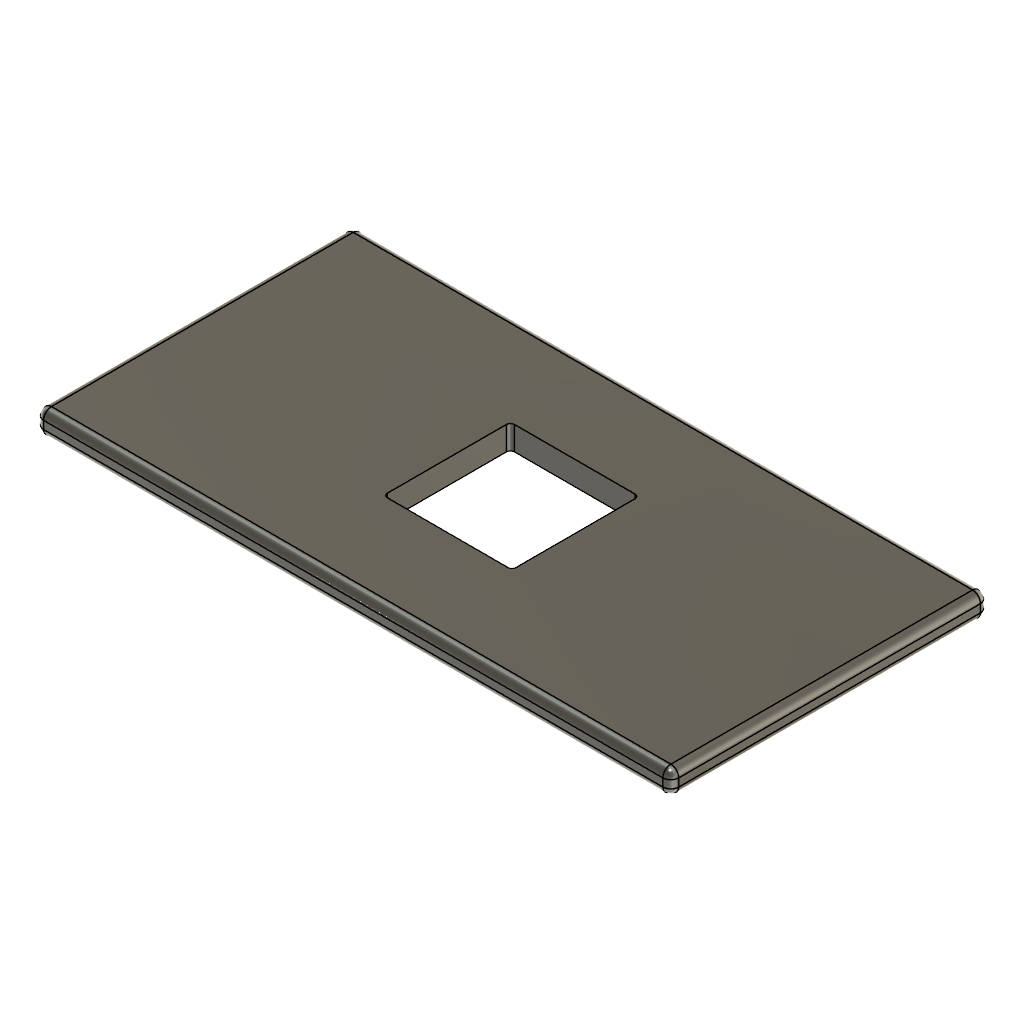
Fan_Holder (Autodesk Fusion 360 design; units mm, degrees)
part number: 2026-09-20-20-59-47-244
Autodesk Fusion 360 part; units mm, degrees
sketch "Sketch1" plane through (0, 0, 0) normal (0, 0, 1) x (1, 0, 0)
  line L0 (-100, 50) -> (300, 50)
  line L1 (300, 50) -> (300, -150)
  line L2 (300, -150) -> (-100, -150)
  line L3 (-100, -150) -> (-100, 50)
  dimension "d1" = 200
  constraint perpendicular L0 L1
  constraint parallel L0 L2
  constraint parallel L1 L3
  constraint horizontal L0
  measures "d1" distance of L0.start L2.end
extrude "Extrude1" add sketch "Sketch1" along normal blind 15
ref_plane "WorkPlane1" through (100, -50, 15) normal (0, 0, 1) x (1, 0, 0)
sketch "Sketch2" plane through (0, 0, 15) normal (0, 0, 1) x (1, 0, 0)
  line L0 (60.5, -9) -> (136.5, -9)
  line L1 (139, -11.5) -> (139, -86.5)
  line L2 (136.5, -89) -> (60.5, -89)
  line L3 (58, -86.5) -> (58, -11.5)
  arc A0 (58, -86.5) -> (60.5, -89) centre (60.5, -86.5) ccw
  arc A1 (136.5, -89) -> (139, -86.5) centre (136.5, -86.5) ccw
  arc A2 (139, -11.5) -> (136.5, -9) centre (136.5, -11.5) ccw
  arc A3 (60.5, -9) -> (58, -11.5) centre (60.5, -11.5) ccw
  dimension "d6" = 2.5
  constraint perpendicular L0 L1
  constraint parallel L0 L2
  constraint parallel L1 L3
  constraint horizontal L0
  constraint tangent L2 A0
  constraint tangent L3 A0
  constraint tangent L1 A1
  constraint tangent L2 A1
  constraint equal A0 A1
  constraint tangent L0 A2
  constraint tangent L1 A2
  constraint equal A0 A2
  constraint tangent L0 A3
  constraint tangent L3 A3
  constraint equal A0 A3
  measures "d6" radius of A0
extrude "Extrude2" cut sketch "Sketch2" against normal blind 70
fillet "Fillet1" radius 5 1 edges at (100, 50, 15)
fillet "Fillet2" radius 5 1 edges at (100, -150, 15)
fillet "Fillet3" radius 5 5 edges at (300, -150, 5) (300, -148.5355, 13.5355) (300, -50, 15) (300, 48.5355, 13.5355) (300, 50, 5)
fillet "Fillet4" radius 5 5 edges at (97.5, 50, 0) (298.5355, 48.5355, 0) (300, -50, 0) (298.5355, -148.5355, 0) (97.5, -150, 0)
fillet "Fillet5" radius 5 8 edges at (-100, -150, 7.5) (-100, -148.5355, 1.4645) (-100, -50, 0) (-100, 48.5355, 1.4645) (-100, 50, 7.5) (-100, 48.5355, 13.5355) (-100, -50, 15) (-100, -148.5355, 13.5355)
